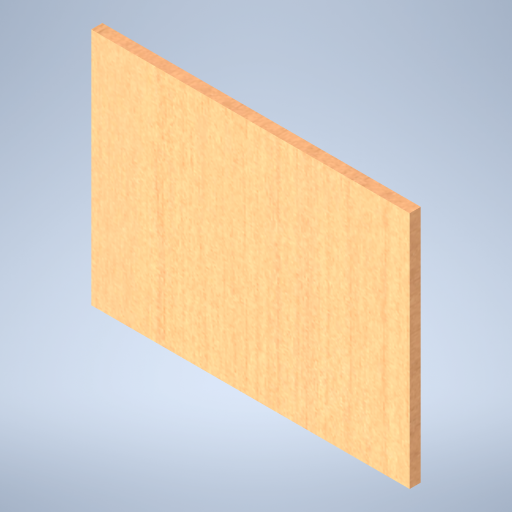
# Autodesk Inventor part: Base
Saved by Autodesk Inventor 2023.1 (Build 271208000, 208)
## iProperties
Created: 2022-10-28
Part Number: Base
Material: MDF Medium Density Fiberboard
Document SubType Name: Modeling
Designer: Daniel Peña
Density: 0.8 g/cm^3
Appearance: Cherry - Natural Low Gloss
Author: Daniel Peña
Autodesk Inventor part; units mm, degrees
ref_plane "YZ Plane" through (0, 0, 0) normal (1, 0, 0) x (0, 1, 0)
ref_plane "XZ Plane" through (0, 0, 0) normal (0, 1, 0) x (-1, 0, 0)
ref_plane "XY Plane" through (0, 0, 0) normal (0, 0, 1) x (1, 0, 0)
sketch "Sketch1" plane through (0, 0, 0) normal (0, 0, 1) x (1, 0, 0)
  line L0 (-100, 75) -> (100, 75)
  line L1 (100, 75) -> (100, -75)
  line L2 (100, -75) -> (-100, -75)
  line L3 (-100, -75) -> (-100, 75)
  point P0 (0, 0)
  dimension "d0" = 200
  dimension "d1" = 150
  dimension "d2" = 75
  dimension "d3" = 100
  constraints: 8 end point, 2 parallel, 1 horizontal, 1 perpendicular
  measures "d0" distance of L1.end L2.end
  measures "d1" distance of L0.end L1.end
  measures "d2" distance from line of L0 point (0, 0)
  measures "d3" distance from line of point (0, 0) L1
extrude "Extrusion1" add sketch "Sketch1" along normal blind 7
equation "\"d2\" = 0.5 * d1"
equation "\"d3\" = 0.5 * d0"
equation "\"d4\" = hMDF"
equation "\"hMDF\" = 7"
body "Solid1"
